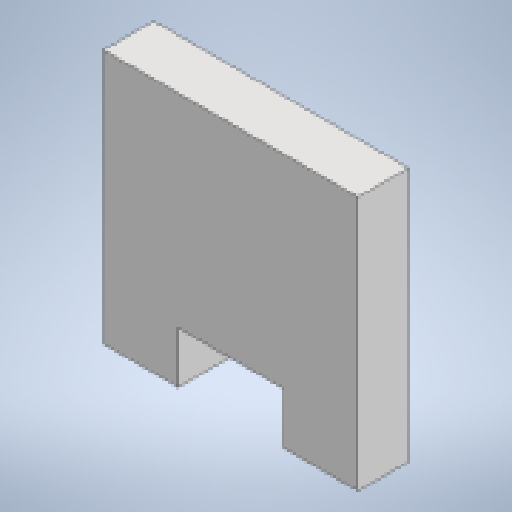
# Autodesk Inventor part: Cemento
Saved by Autodesk Inventor 2024 (Build 280153000, 153)
## iProperties
Created: 2024-07-16
Part Number: Cemento
Material: Genérico
Document SubType Name: Modeling
Designer: sergi
Density: 1 g/cm^3
Appearance: Valor por defecto
Author: sergi
Autodesk Inventor part; units mm, degrees
ref_plane "YZ Plane" through (0, 0, 0) normal (1, 0, 0) x (0, 1, 0)
ref_plane "XZ Plane" through (0, 0, 0) normal (0, 1, 0) x (-1, 0, 0)
ref_plane "XY Plane" through (0, 0, 0) normal (0, 0, 1) x (1, 0, 0)
sketch "Boceto1" plane through (0, 0, 0) normal (0, 0, 1) x (1, 0, 0)
  line L0 (40.8, -59.2) -> (-40.8, -59.2) projected
  line L1 (40.8, -79.7) -> (40.8, -59.2) projected
  line L2 (99.2, -99.2) -> (58.3, -99.2) projected
  line L3 (99.2, -58.3) -> (99.2, -99.2) projected
  line L4 (58.3, 99.2) -> (99.2, 99.2) projected
  line L5 (-99.2, 58.3) -> (-99.2, 99.2) projected
  line L6 (-58.3, -99.2) -> (-99.2, -99.2) projected
  line L7 (-40.8, -59.2) -> (-40.8, -79.7) projected
  line L8 (-40.8, -79.7) -> (-58.3, -79.7) projected
  line L9 (58.3, -79.7) -> (40.8, -79.7) projected
  line L10 (58.3, -99.2) -> (58.3, -79.7) projected
  line L11 (79.7, -58.3) -> (99.2, -58.3) projected
  line L12 (79.7, -41.7) -> (79.7, -58.3) projected
  line L13 (99.2, -41.7) -> (79.7, -41.7) projected
  line L14 (99.2, 41.7) -> (99.2, -41.7) projected
  line L15 (79.7, 41.7) -> (99.2, 41.7) projected
  line L16 (79.7, 58.3) -> (79.7, 41.7) projected
  line L17 (99.2, 58.3) -> (79.7, 58.3) projected
  line L18 (99.2, 99.2) -> (99.2, 58.3) projected
  line L19 (58.3, 79.7) -> (58.3, 99.2) projected
  line L20 (41.7, 79.7) -> (58.3, 79.7) projected
  line L21 (41.7, 99.2) -> (41.7, 79.7) projected
  line L22 (-41.7, 99.2) -> (41.7, 99.2) projected
  line L23 (-41.7, 79.7) -> (-41.7, 99.2) projected
  line L24 (-58.3, 79.7) -> (-41.7, 79.7) projected
  line L25 (-58.3, 99.2) -> (-58.3, 79.7) projected
  line L26 (-99.2, 99.2) -> (-58.3, 99.2) projected
  line L27 (-79.7, 58.3) -> (-99.2, 58.3) projected
  line L28 (-79.7, 41.7) -> (-79.7, 58.3) projected
  line L29 (-99.2, 41.7) -> (-79.7, 41.7) projected
  line L30 (-99.2, -41.7) -> (-99.2, 41.7) projected
  line L31 (-79.7, -41.7) -> (-99.2, -41.7) projected
  line L32 (-79.7, -58.3) -> (-79.7, -41.7) projected
  line L33 (-99.2, -58.3) -> (-79.7, -58.3) projected
  line L34 (-99.2, -99.2) -> (-99.2, -58.3) projected
  line L35 (-58.3, -79.7) -> (-58.3, -99.2) projected
  point P0 (0, 0)
ref_plane "Plano de trabajo1" through (-100, -100, 39.2) normal (0, 0, 1) x (1, 0, 0)
extrude "Extrusión1" add sketch "Boceto1" along normal up to surface (39.2 mm away)
